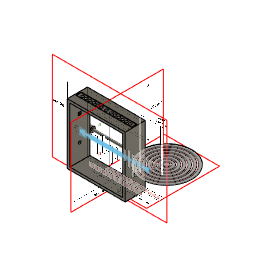
water-drop-mechanism-11052020 (Autodesk Fusion 360 design; units mm, degrees)
Autodesk Fusion 360 part; units mm, degrees
note: some values were not read from the file. Set by a fixed rule: which sketch regions a step uses.
sketch "body extrude" plane through (0, 0, 0) normal (0, 1, 0) x (1, 0, 0) in component "body"
  line L0 (66, -150) -> (-39.1, -150)
  line L1 (-39.1, -150) -> (-39.1, -39.7)
  line L2 (-39.1, -39.7) -> (66, -39.7)
  line L3 (66, -39.7) -> (66, -150)
  line L4 (-44.1, -34.7) -> (71, -34.7)
  line L5 (71, -34.7) -> (71, -155)
  line L6 (71, -155) -> (-44.1, -155)
  line L7 (-44.1, -155) -> (-44.1, -34.7)
  constraint horizontal L0
  constraint vertical L1
  constraint horizontal L2
  constraint vertical L3
  constraint horizontal L4
  constraint vertical L5
  constraint horizontal L6
  constraint vertical L7
extrude "Extrude1" add sketch "body extrude" against normal blind 40 makes body 1 in component "body"
sketch "body side and interior holes" plane through (-44.1, 0, 0) normal (-1, 0, 0) x (0, -1, 0) in component "body"
  line L0 (0, 155) -> (0, 34.7)
  line L1 (0, 34.7) -> (40, 34.7)
  line L2 (40, 34.7) -> (40, 155)
  line L3 (40, 155) -> (0, 155)
  line L4 (17.5, 75) -> (23, 75)
  line L5 (23, 75) -> (23, 69.5)
  line L6 (23, 69.5) -> (17.5, 69.5)
  line L7 (17.5, 69.5) -> (17.5, 75)
  line L8 (17.5, 125) -> (23, 125)
  line L9 (23, 125) -> (23, 119.5)
  line L10 (23, 119.5) -> (17.5, 119.5)
  line L11 (17.5, 119.5) -> (17.5, 125)
  circle A0 centre (20.25, 72.25) radius 2.75
  dimension "d3" = 5.5
  dimension "d4" = 5.5
  constraint horizontal L4
  constraint vertical L5
  constraint horizontal L6
  constraint vertical L7
  constraint horizontal L8
  constraint vertical L9
  constraint horizontal L10
  constraint vertical L11
  constraint tangent L5 A0
  measures "d3" distance of L8.start L8.end
  measures "d4" distance of L8.start L10.end
extrude "Extrude2" cut sketch "body side and interior holes" against normal blind 145 contours A0 bodies 1 in component "body"
extrude "Extrude3" cut sketch "body side and interior holes" along normal blind -112.5 and the other way blind 2.5 contours L8 L9 L10 L11 bodies 1 in component "body"
sketch "body top holes" plane through (0, 0, 155) normal (0, 0, 1) x (-1, 0, 0) in component "body"
  line L0 (-71, 0) -> (44.1, 0)
  line L1 (44.1, 0) -> (44.1, 40)
  line L2 (44.1, 40) -> (-71, 40)
  line L3 (-71, 40) -> (-71, 0)
  line L4 (41.7114, 14.6402) -> (-68.5, 14.6402)
  line L5 (-68.5, 14.6402) -> (-68.5, 25.2)
  line L6 (-68.5, 25.2) -> (41.7114, 25.2)
  line L7 (41.7114, 25.2) -> (41.7114, 14.6402)
  line L8 (-58, 17) -> (-63.5, 17)
  line L9 (-63.5, 17) -> (-63.5, 22.5)
  line L10 (-63.5, 22.5) -> (-58, 22.5)
  line L11 (-58, 22.5) -> (-58, 17)
  line L12 (-56, 17) -> (-50.5, 17)
  line L13 (-50.5, 17) -> (-50.5, 22.5)
  line L14 (-50.5, 22.5) -> (-56, 22.5)
  line L15 (-56, 22.5) -> (-56, 17)
  line L16 (-48.5, 17) -> (-43, 17)
  line L17 (-43, 17) -> (-43, 22.5)
  line L18 (-43, 22.5) -> (-48.5, 22.5)
  line L19 (-48.5, 22.5) -> (-48.5, 17)
  line L20 (-20.5, 17) -> (-26, 17)
  line L21 (-26, 17) -> (-26, 22.5)
  line L22 (-26, 22.5) -> (-20.5, 22.5)
  line L23 (-20.5, 22.5) -> (-20.5, 17)
  line L24 (-28, 17) -> (-33.5, 17)
  line L25 (-33.5, 17) -> (-33.5, 22.5)
  line L26 (-33.5, 22.5) -> (-28, 22.5)
  line L27 (-28, 22.5) -> (-28, 17)
  line L28 (-35.5, 17) -> (-41, 17)
  line L29 (-41, 17) -> (-41, 22.5)
  line L30 (-41, 22.5) -> (-35.5, 22.5)
  line L31 (-35.5, 22.5) -> (-35.5, 17)
  line L32 (-13.3943, 14.6402) -> (-13.3943, 25.2) construction
  line L33 (-20.5, 19.75) -> (-13.5, 19.75) construction
  line L34 (-13.5, 19.75) -> (-16.25, 19.75)
  line L35 (-16.25, 19.75) -> (-16.25, 17)
  line L36 (-16.25, 17) -> (-13.5, 17)
  line L37 (-13.5, 17) -> (-13.5, 19.75)
  line L38 (-16.25, 17) -> (-10.75, 17)
  line L39 (-10.75, 17) -> (-10.75, 22.5)
  line L40 (-10.75, 22.5) -> (-16.25, 22.5)
  line L41 (-16.25, 22.5) -> (-16.25, 17)
  circle A0 centre (-23.25, 19.75) radius 2.75
  circle A1 centre (-30.75, 19.75) radius 2.75
  circle A2 centre (-38.25, 19.75) radius 2.75
  circle A3 centre (-45.75, 19.75) radius 2.75
  circle A4 centre (-53.25, 19.75) radius 2.75
  circle A5 centre (-60.75, 19.75) radius 2.75
  line L42 (6.7114, 17) -> (6.7114, 22.5)
  line L43 (23.7114, 17) -> (23.7114, 22.5)
  line L44 (23.7114, 22.5) -> (29.2114, 22.5)
  line L45 (21.7114, 17) -> (16.2114, 17)
  circle A6 centre (26.4614, 19.75) radius 2.75
  circle A7 centre (18.9614, 19.75) radius 2.75
  line L46 (14.2114, 17) -> (14.2114, 22.5)
  line L47 (36.7114, 17) -> (36.7114, 22.5)
  line L48 (21.7114, 22.5) -> (21.7114, 17)
  line L49 (-6.2886, 17) -> (-0.7886, 17)
  line L50 (-6.2886, 22.5) -> (-6.2886, 17)
  circle A8 centre (3.9614, 19.75) radius 2.75
  line L51 (31.2114, 22.5) -> (31.2114, 17)
  line L52 (16.2114, 22.5) -> (21.7114, 22.5)
  line L53 (36.7114, 22.5) -> (31.2114, 22.5)
  line L54 (1.2114, 22.5) -> (1.2114, 17)
  line L55 (8.7114, 22.5) -> (8.7114, 17)
  circle A9 centre (-3.5386, 19.75) radius 2.75
  line L56 (14.2114, 22.5) -> (8.7114, 22.5)
  line L57 (16.2114, 17) -> (16.2114, 22.5)
  line L58 (29.2114, 17) -> (23.7114, 17)
  line L59 (1.2114, 17) -> (6.7114, 17)
  circle A10 centre (33.9614, 19.75) radius 2.75
  line L60 (29.2114, 22.5) -> (29.2114, 17)
  line L61 (-0.7886, 17) -> (-0.7886, 22.5)
  circle A11 centre (11.4614, 19.75) radius 2.75
  line L62 (6.7114, 22.5) -> (1.2114, 22.5)
  line L63 (31.2114, 17) -> (36.7114, 17)
  line L64 (-0.7886, 22.5) -> (-6.2886, 22.5)
  line L65 (8.7114, 17) -> (14.2114, 17)
  circle A12 centre (-13.5, 19.75) radius 2.75
  point P0 (-6.2886, 19.75)
  constraint horizontal L4
  constraint vertical L5
  constraint horizontal L6
  constraint vertical L7
  constraint horizontal L8
  constraint vertical L9
  constraint horizontal L10
  constraint vertical L11
  constraint horizontal L12
  constraint vertical L13
  constraint horizontal L14
  constraint vertical L15
  constraint horizontal L16
  constraint vertical L17
  constraint horizontal L18
  constraint vertical L19
  constraint horizontal L20
  constraint vertical L21
  constraint horizontal L22
  constraint vertical L23
  constraint horizontal L24
  constraint vertical L25
  constraint horizontal L26
  constraint vertical L27
  constraint horizontal L28
  constraint vertical L29
  constraint horizontal L30
  constraint vertical L31
  constraint midpoint L4 L32.start
  constraint midpoint L6 L32.end
  constraint midpoint L23 L33.start
  constraint perpendicular L23 L33
  constraint horizontal L34
  constraint vertical L35
  constraint horizontal L36
  constraint vertical L37
  constraint horizontal L38
  constraint vertical L39
  constraint horizontal L40
  constraint vertical L41
  constraint tangent L21 A0
  constraint coincident L33.start A0
  constraint tangent L25 A1
  constraint tangent L29 A2
  constraint tangent L19 A3
  constraint tangent L15 A4
  constraint tangent L9 A5
  constraint symmetric L8.start L32 L51.end
  constraint symmetric L8.end L32 L47.start
  constraint symmetric L9.end L32 L47.end
  constraint symmetric L10.end L32 L51.start
  constraint symmetric L12.start L32 L58.start
  constraint symmetric L12.end L32 L43.start
  constraint symmetric L13.end L32 L43.end
  constraint symmetric L14.end L32 L44.end
  constraint symmetric L16.start L32 L45.start
  constraint symmetric L16.end L32 L45.end
  constraint symmetric L17.end L32 L52.start
  constraint symmetric L18.end L32 L48.start
  constraint symmetric L20.start L32 L49.start
  constraint symmetric L20.end L32 L49.end
  constraint symmetric L21.end L32 L61.end
  constraint symmetric L22.end L32 L50.start
  constraint symmetric L24.start L32 L54.end
  constraint symmetric L24.end L32 L42.start
  constraint symmetric L25.end L32 L42.end
  constraint symmetric L26.end L32 L54.start
  constraint symmetric L28.start L32 L55.end
  constraint symmetric L28.end L32 L46.start
  constraint symmetric L29.end L32 L46.end
  constraint symmetric L30.end L32 L55.start
  constraint symmetric L32 L33.start P0
  constraint symmetric L32 A0 A9
  constraint symmetric L32 A1 A8
  constraint symmetric L32 A2 A11
  constraint symmetric L32 A3 A7
  constraint symmetric L32 A4 A6
  constraint symmetric L32 A5 A10
  constraint coincident L34.end A12
  constraint tangent L35 A12
extrude "Extrude5" cut sketch "body top holes" against normal blind 1 contours L4 L5 L6 L7 | L8 L11 A5 | L8 L9 A5 | L10 L11 A5 | L9 L10 A5 | L12 L15 A4 | L12 L13 A4 | L14 L15 A4 | L13 L14 A4 | L16 L19 A3 | L16 L17 A3 | L18 L19 A3 | L17 L18 A3 | L20 L23 A0 | L20 L21 A0 | L22 L23 A0 | L21 L22 A0 | L24 L27 A1 | L24 L25 A1 | L26 L27 A1 | L25 L26 A1 | L28 L31 A2 | L28 L29 A2 | L30 L31 A2 | L29 L30 A2 | L35 L36 L38 L41 A12 | L40 L41 A12 | L38 L39 A12 | L39 L40 A12 | L42 A8 L59 | L42 A8 L62 | A8 L54 L59 | A8 L54 L62 | L43 A6 L58 | L43 L44 A6 | A6 L58 L60 | L44 A6 L60 | L45 A7 L48 | L45 A7 L57 | A7 L48 L52 | A7 L52 L57 | L46 A11 L65 | L46 L56 A11 | L55 A11 L65 | L55 L56 A11 | L47 A10 L63 | L47 L53 A10 | L51 A10 L63 | L51 L53 A10 | L49 L50 A9 | L49 A9 L61 | L50 A9 L64 | A9 L61 L64 bodies 1 in component "body"
extrude "Extrude4" cut sketch "body top holes" against normal blind 30 contours A5 | A4 | A3 | A0 | A1 | A2 | L34 L37 A12 | L34 L37 A12 | A8 | A6 | A7 | A11 | A10 | A9 bodies 1 in component "body"
sketch "circles" plane through (0, 0, 0) normal (0, 0, 1) x (1, 0, 0) in component "circles"
  circle A0 centre (13.5, 100) radius 5
  circle A1 centre (13.5, 100) radius 7.5
  circle A2 centre (13.5, 100) radius 12.5
  circle A3 centre (13.5, 100) radius 14.9848
  circle A4 centre (13.5, 100) radius 19.9601
  circle A5 centre (13.5, 100) radius 22.5
  circle A6 centre (13.5, 100) radius 27.5
  circle A7 centre (13.5, 100) radius 29.9983
  circle A8 centre (13.5, 100) radius 34.9045
  circle A9 centre (13.5, 100) radius 37.5
  circle A10 centre (13.5, 100) radius 42.5
  circle A11 centre (13.5, 100) radius 45
  circle A12 centre (13.5, 100) radius 50.0143
  constraint concentric A0 A1
  constraint concentric A0 A2
  constraint concentric A1 A3
  constraint concentric A3 A4
  constraint concentric A4 A5
  constraint concentric A0 A6
  constraint concentric A2 A7
  constraint concentric A4 A8
  constraint concentric A2 A9
  constraint concentric A5 A10
  constraint concentric A3 A11
  constraint concentric A4 A12
extrude "Extrude1'" add sketch "circles" along normal blind 1 separate body makes body 2 at (46.6392, 98.2659, 0) makes body 3 at (13.1291, 103.0712, 0) makes body 4 at (39.2309, 98.6338, 0) makes body 5 at (54.0355, 96.0255, 0) makes body 6 at (24.2868, 99.379, 0) makes body 7 at (31.6716, 98.2639, 0) makes body 8 at (61.4891, 95.2796, 0) in component "circles"
sketch "moving rod" plane through (0, 0, 0) normal (0, 1, 0) x (1, 0, 0) in component "moving rod"
  line L0 (-55, -75) -> (75.8973, -75)
  line L1 (75.8973, -75) -> (75.8973, -69.6638)
  line L2 (75.8973, -69.6638) -> (-55, -69.6638)
  line L3 (-55, -69.6638) -> (-55, -75)
  line L4 (-55, -72.3319) -> (75.8973, -72.3319)
  line L5 (-48.5, -77.5) -> (-58.5, -77.5)
  line L6 (-58.5, -77.5) -> (-58.5, -66.5)
  line L7 (-58.5, -66.5) -> (-48.5, -66.5)
  line L8 (-48.5, -66.5) -> (-48.5, -77.5)
  line L9 (-55, -72.3319) -> (-58.5, -72.3319)
  constraint horizontal L0
  constraint vertical L1
  constraint horizontal L2
  constraint vertical L3
  constraint midpoint L3 L4.start
  constraint midpoint L1 L4.end
  constraint horizontal L5
  constraint vertical L6
  constraint horizontal L7
  constraint vertical L8
  constraint coincident L6 L9.end
  constraint perpendicular L6 L9
revolve "Revolve1" add sketch "moving rod" angle 360 about axis through (-55, 0, 72.3319) along (1, 0, 0) separate body contours L0 L3 L4 L8 | L0 L1 L4 L8 makes body 9 in component "moving rod"
revolve "Revolve2" add sketch "moving rod" angle 360 about axis through (-55, 0, 72.3319) along (-1, 0, 0) contours L0 L3 L4 L8 | L0 L3 L5 L6 L8 L9 bodies 9 in component "moving rod"
move_body "Move1" bodies 9 to x (1, 0, 0) y (0, 1, 0) z (0, 0, 1) at (0, 15, 0) in component "moving rod"
move_face "OffsetFaces1" offset -0.3 1 faces at (-7.0342, 17.5292, 71.4822) on bodies 9 in component "moving rod"
component "body" placed x (1, 0, 0) y (0, 1, 0) z (0, 0, 1) at (0, 0, 0)
component "circles" placed x (1, 0, 0) y (0, 1, 0) z (0, 0, 1) at (0, 0, 0)
component "moving rod" placed x (1, 0, 0) y (0, 1, 0) z (0, 0, 1) at (0, 0, 0)
component "support rods" placed x (1, 0, 0) y (0, 1, 0) z (0, 0, 1) at (0, 0, 0)
named bodies: "body", "3_circle", "7_circle", "4_circle", "2_circle", "6_circle", "5_circle", "1_circle", "moving rod"
